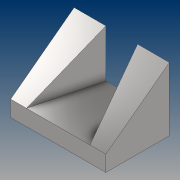
# Autodesk Inventor part: 9
Saved by Autodesk Inventor 2020.2 (Build 242310000, 310)
## iProperties
Created: 2020-09-17
Part Number: 9
Material: 鋼、碳鋼
Document SubType Name: Modeling
Designer: user
Density: 7.85 g/cm^3
Appearance: 半拋光
Mass: 345.4 g
Surface Area: 107.369 cm^2
Volume: 44 cm^3
Author: user
Autodesk Inventor part; units mm, degrees
ref_plane "YZ Plane" through (0, 0, 0) normal (1, 0, 0) x (0, 1, 0)
ref_plane "XZ Plane" through (0, 0, 0) normal (0, 1, 0) x (-1, 0, 0)
sketch "草圖1" plane through (0, 0, 0) normal (0, 1, 0) x (-1, 0, 0)
  line L0 (-30, 20) -> (30, 20)
  line L1 (30, 20) -> (30, -20)
  line L2 (30, -20) -> (-30, -20)
  line L3 (-30, -20) -> (-30, 20)
  line L4 (-30, 20) -> (30, -20) construction
  line L5 (30, 20) -> (-30, -20) construction
  point P0 (0, 0)
  point P1 (0, 0)
  point P2 (0, 0)
  dimension "d0" = 60
  dimension "d1" = 40
  constraints: 12 end point, 3 midpoint, 2 parallel, 1 coincident, 1 horizontal, 1 perpendicular
  measures "d0" distance of L1.end L2.end
  measures "d1" distance of L2.end L0.start
extrude "擠出1" add sketch "草圖1" along normal blind 40
sketch "草圖2" plane through (30, 0, 20) normal (1, 0, 0) x (0, 0, -1)
  line L0 (0, 0) -> (0, 40) projected
  line L1 (0, 40) -> (40, 40) projected
  line L2 (40, 40) -> (40, 0) projected
  line L3 (40, 0) -> (0, 0) projected
  line L4 (0, 40) -> (40, 40) projected
  line L5 (40, 40) -> (0, 10)
  point P0 (20, 0)
  dimension "d4" = 10
  constraints: 2 end point, 1 point on line
  measures "d4" distance from line of L5.end L3
extrude "擠出2" cut sketch "草圖2" against normal through all contours L0 L1 L5
ref_plane "工作平面1" through (30, 10, 20) normal (0, -1, 0) x (1, 0, 0)
sketch "草圖3" plane through (30, 10, 20) normal (0, -1, 0) x (1, 0, 0)
  line L0 (-60, 0) -> (0, 0) projected
  line L1 (0, 0) -> (0, -40) projected
  line L2 (0, -40) -> (-60, -40) projected
  line L3 (-60, -40) -> (-60, 0) projected
  line L4 (-60, 0) -> (0, 0) projected
  line L5 (-50, 0) -> (-40, -40)
  line L6 (0, -40) -> (-60, -40) projected
  line L7 (-20, -40) -> (-10, 0)
  point P0 (-30, -20)
  point P1 (-10, 0)
  point P2 (-50, 0)
  dimension "d7" = 10
  dimension "d8" = 20
  dimension "d9" = 20
  dimension "d10" = 40
  constraints: 4 end point, 4 point on line
  measures "d7" horizontal distance of L5.end point (-30, -20)
  measures "d8" distance of L7.start L5.end
  measures "d9" horizontal distance of point (-30, -20) L5.start
  measures "d10" distance of L7.end L5.start
extrude "擠出3" cut sketch "草圖3" against normal blind 53 contours L0 L7 L2 L5
